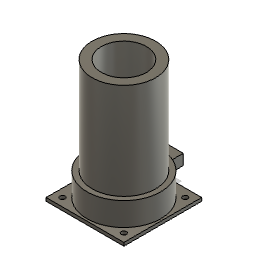
PiFinder_DIY (Autodesk Fusion 360 archive; units mm, degrees)
design "RPI HQ Cam"
Autodesk Fusion 360 part; units mm, degrees
sketch "camera_dimensions" plane through (0, 0, 0) normal (0, 1, 0) x (1, 0, 0)
  line L0 (19, -19) -> (-19, -19)
  line L1 (-19, -19) -> (-19, 19)
  line L2 (-19, 19) -> (19, 19)
  line L3 (19, 19) -> (19, -19)
  line L4 (19, -19) -> (-19, 19) construction
  line L5 (-19, -19) -> (19, 19) construction
  circle A0 centre (-15, 15) radius 1.25
  circle A1 centre (15, 15) radius 1.25
  circle A2 centre (-15, -15) radius 1.25
  circle A3 centre (15, -15) radius 1.25
  circle A4 centre (0, 0) radius 18
  circle A5 centre (0, 0) radius 15.5
  circle A6 centre (0, 0) radius 11
  line L6 (-6, 16) -> (6, 16)
  line L7 (6, 16) -> (6, 23)
  line L8 (6, 23) -> (-6, 23)
  line L9 (-6, 23) -> (-6, 16)
  line L10 (0, 30) -> (0, -25) construction
  dimension "d1" = 38
  dimension "d2" = 38
  dimension "d3" = 2.5
  dimension "d4" = 4
  dimension "d5" = 4
  dimension "d6" = 2.5
  dimension "d7" = 2.5
  dimension "d8" = 2.5
  dimension "d9" = 4
  dimension "d10" = 4
  dimension "d11" = 4
  dimension "d12" = 4
  dimension "d13" = 4
  dimension "d14" = 4
  dimension "d15" = 36
  dimension "d16" = 31
  dimension "d17" = 22
  dimension "d18" = 12
  constraint horizontal L0
  constraint perpendicular L0 L1
  constraint parallel L0 L2
  constraint parallel L1 L3
  constraint coincident L4 A4.centre
  constraint coincident L5 A4.centre
  constraint coincident A4.centre A5.centre
  constraint horizontal L6
  constraint vertical L7
  constraint horizontal L8
  constraint vertical L9
  constraint perpendicular L0 L10
  constraint symmetric L7 L9 L10
  measures "d1" distance of L1.end L2.end
  measures "d2" distance of L0.end L1.end
  measures "d3" diameter of A0
  measures "d4" distance of L1 A0.centre
  measures "d5" distance of L2 A0.centre
  measures "d6" diameter of A1
  measures "d7" diameter of A2
  measures "d8" diameter of A3
  measures "d9" distance of L3 A3.centre
  measures "d10" distance of L0 A3.centre
  measures "d11" distance of L2 A1.centre
  measures "d12" distance of L3 A1.centre
  measures "d13" distance of L0 A2.centre
  measures "d14" distance of L1 A2.centre
  measures "d15" diameter of A4
  measures "d16" diameter of A5
  measures "d17" diameter of A6
  measures "d18" distance of L7.end L8.end
extrude "Extrude1" add sketch "camera_dimensions" along normal blind 1.6 contours L0 L1 L2 L3 A4 L7 L9 | L2 A4 L7 L9 | A4 L6 L7 L9 | A4 L6 L7 L9 | A5 | A6
extrude "Extrude2" add sketch "camera_dimensions" along normal blind 11.4 from surface at 1.6 contours A4 L6 L7 L9 | A4 L6 L7 L9 | A5
extrude "Extrude3" add sketch "camera_dimensions" along normal blind 60 contours A5
extrude "Extrude4" add sketch "camera_dimensions" along normal blind 5.2 from surface at 6.6 contours L2 A4 L7 L9 | L2 L7 L8 L9
named bodies: "PiHQCam_mockup"
